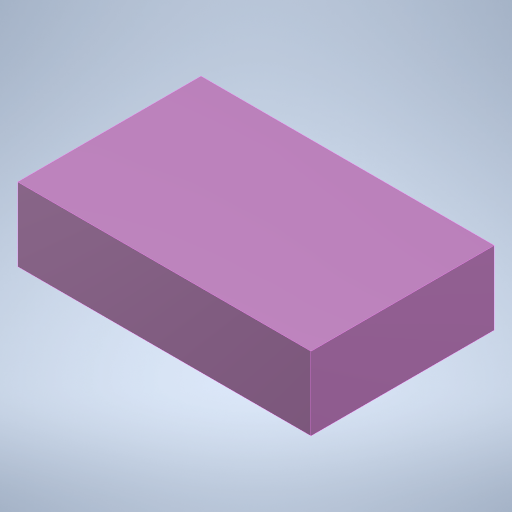
# Autodesk Inventor part: NYAK_sacc
Saved by Autodesk Inventor 2023 (Build 270158000, 158)
## iProperties
Created: 2023-04-27
Part Number: NYAK_sacc
Material: Generic
Document SubType Name: Modeling
Designer: nagyb
Density: 1 g/cm^3
Appearance: Smooth - Purple
Author: nagyb
Autodesk Inventor part; units mm, degrees
ref_plane "YZ Plane" through (0, 0, 0) normal (1, 0, 0) x (0, 1, 0)
ref_plane "XZ Plane" through (0, 0, 0) normal (0, 1, 0) x (-1, 0, 0)
ref_plane "XY Plane" through (0, 0, 0) normal (0, 0, 1) x (1, 0, 0)
sketch "Sketch1" plane through (0, 0, 0) normal (0, 1, 0) x (-1, 0, 0)
  line L0 (-80, -50) -> (80, -50)
  line L1 (80, -50) -> (80, 50)
  line L2 (80, 50) -> (-80, 50)
  line L3 (-80, 50) -> (-80, -50)
  line L4 (-80, -50) -> (80, 50) construction
  line L5 (80, -50) -> (-80, 50) construction
  point P0 (0, 0)
  dimension "d0" = 160
  dimension "d1" = 100
  constraints: 12 end point, 2 midpoint, 2 parallel, 1 horizontal, 1 perpendicular
  measures "d0" distance of L1.end L2.end
  measures "d1" distance of L0.end L1.end
extrude "Extrusion1" add sketch "Sketch1" along normal blind 40
body "Solid1"
